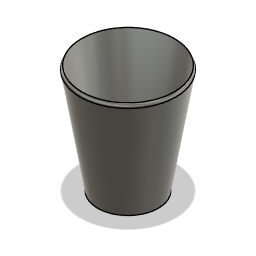
wzken爆改熔岩灯2顶盖刻字 (Autodesk Fusion 360 design; units mm, degrees)
Autodesk Fusion 360 part; units mm, degrees
(part 1 of 7)
sketch "草图1" plane through (0, 0, 0) normal (0, 1, 0) x (1, 0, 0)
  circle A0 centre (0, 0) radius 22.5
  circle A1 centre (0, 0) radius 13.75
  circle A2 centre (0, 0) radius 14.75
  circle A3 centre (0, 0) radius 23.5
  spline S0 degree 3 poles (1.8081, 3.6652) (1.7986, 3.6895) (1.7856, 3.712) (1.7795, 3.7138) knots 0 0 0 0 1 1 1 1
  dimension "d1" = 45
  dimension "d2" = 27.5
  dimension "d3" = 29.5
  dimension "d4" = 47
  constraint coincident A0.centre A1.centre
  constraint concentric A0 A1
  constraint concentric A0 A2
  constraint concentric A1 A3
  measures "d1" diameter of A0
  measures "d2" diameter of A1
  measures "d3" diameter of A2
  measures "d4" diameter of A3
extrude "拉伸1" add sketch "草图1" along normal blind 53 draft 9.4 contours A2
extrude "拉伸2" cut sketch "草图1" along normal blind 53 draft 9.4 contours A1
extrude "拉伸3" add sketch "草图1" along normal blind 2 draft 9.4 contours A1
fillet "圆角1" radius 2 1 edges at (-21.9322, 53, -8.5067)
sketch "草图2" plane through (0, 2, 0) normal (0, 1, 0) x (-1, 0, 0)
  circle A0 centre (0, 0) radius 14.0811
  line L0 (27.3607, -10.0098) -> (27.3607, 8.4871)
  line L1 (27.3607, 8.4871) -> (-0.3846, 8.4871)
  line L2 (-0.3846, 8.4871) -> (-28.1299, 8.4871)
  line L3 (-28.1299, 8.4871) -> (-28.1299, -10.0098)
  line L4 (-28.1299, -10.0098) -> (-28.1299, -28.5067)
  line L5 (-28.1299, -28.5067) -> (-0.3846, -28.5067)
  line L6 (-0.3846, -28.5067) -> (27.3607, -28.5067)
  line L7 (27.3607, -28.5067) -> (27.3607, -10.0098)
  spline S0 degree 3 poles (-1.1505, -12.3075) (-1.1794, -12.2641) (-1.1938, -11.6572) (-1.1866, -10.9708) knots 0 0 0 0 1 1 1 1
  line L8 (-1.1866, -10.9708) -> (-1.1721, -9.7136)
  line L9 (-1.1721, -9.7136) -> (-1.3455, -9.8292)
  spline S1 degree 3 poles (-1.3455, -9.8292) (-1.4395, -9.887) (-1.6707, -10.1326) (-1.8513, -10.3711) knots 0 0 0 0 1 1 1 1
  line L10 (-1.8513, -10.3711) -> (-2.1837, -10.7974)
  line L11 (-2.1837, -10.7974) -> (-1.9236, -10.819)
  spline S2 degree 3 poles (-1.9236, -10.819) (-1.7791, -10.8335) (-1.649, -10.8841) (-1.6273, -10.9347) knots 0 0 0 0 1 1 1 1
  spline S3 degree 3 poles (-1.6273, -10.9347) (-1.6056, -10.9997) (-1.7502, -11.0214) (-2.1837, -11.0214) knots 0 0 0 0 1 1 1 1
  spline S4 degree 3 poles (-2.1837, -11.0214) (-2.5088, -11.0214) (-2.7689, -10.9925) (-2.7689, -10.9563) knots 0 0 0 0 1 1 1 1
  spline S5 degree 3 poles (-2.7689, -10.9563) (-2.7689, -10.9202) (-2.5883, -10.7323) (-2.3715, -10.5517) knots 0 0 0 0 1 1 1 1
  spline S6 degree 3 poles (-2.3715, -10.5517) (-2.1548, -10.3639) (-1.9958, -10.1832) (-2.0175, -10.1471) knots 0 0 0 0 1 1 1 1
  spline S7 degree 3 poles (-2.0175, -10.1471) (-2.0392, -10.111) (-2.0175, -10.0893) (-1.9669, -10.0965) knots 0 0 0 0 1 1 1 1
  spline S8 degree 3 poles (-1.9669, -10.0965) (-1.9163, -10.111) (-1.8296, -10.0315) (-1.7646, -9.9231) knots 0 0 0 0 1 1 1 1
  spline S9 degree 3 poles (-1.7646, -9.9231) (-1.649, -9.728) (-1.649, -9.7208) (-2.1186, -9.2439) knots 0 0 0 0 1 1 1 1
  spline S10 degree 3 poles (-2.1186, -9.2439) (-2.3788, -8.9838) (-2.7183, -8.702) (-2.8773, -8.6153) knots 0 0 0 0 1 1 1 1
  line L12 (-2.8773, -8.6153) -> (-3.1663, -8.4564)
  line L13 (-3.1663, -8.4564) -> (-2.5955, -8.4347)
  spline S11 degree 3 poles (-2.5955, -8.4347) (-1.9814, -8.413) (-1.9091, -8.4347) (-2.0392, -8.5936) knots 0 0 0 0 1 1 1 1
  spline S12 degree 3 poles (-2.0392, -8.5936) (-2.1042, -8.6731) (-2.0319, -8.7743) (-1.6707, -9.1283) knots 0 0 0 0 1 1 1 1
  line L14 (-1.6707, -9.1283) -> (-1.2155, -9.5691)
  line L15 (-1.2155, -9.5691) -> (-1.1721, -9.3306)
  spline S13 degree 3 poles (-1.1721, -9.3306) (-1.0999, -8.8899) (-1.1721, -8.5936) (-1.3817, -8.5142) knots 0 0 0 0 1 1 1 1
  spline S14 degree 3 poles (-1.3817, -8.5142) (-1.5478, -8.4491) (-1.4756, -8.4347) (-0.9843, -8.4275) knots 0 0 0 0 1 1 1 1
  spline S15 degree 3 poles (-0.9843, -8.4275) (-0.399, -8.4202) (-0.1967, -8.4997) (-0.5652, -8.5936) knots 0 0 0 0 1 1 1 1
  line L16 (-0.5652, -8.5936) -> (-0.7458, -8.637)
  line L17 (-0.7458, -8.637) -> (-0.7314, -10.1326)
  line L18 (-0.7314, -10.1326) -> (-0.7097, -11.6283)
  line L19 (-0.7097, -11.6283) -> (-0.4279, -11.7078)
  spline S16 degree 3 poles (-0.4279, -11.7078) (-0.1245, -11.7945) (-0.1389, -11.8378) (-0.4929, -11.9173) knots 0 0 0 0 1 1 1 1
  spline S17 degree 3 poles (-0.4929, -11.9173) (-0.7675, -11.9896) (-0.8903, -12.0907) (-0.8903, -12.2569) knots 0 0 0 0 1 1 1 1
  spline S18 degree 3 poles (-0.8903, -12.2569) (-0.8903, -12.4086) (-1.071, -12.4447) (-1.1505, -12.3075) knots 0 0 0 0 1 1 1 1
  spline S19 degree 3 poles (5.5836, -11.6066) (5.5619, -11.5705) (5.6052, -11.5271) (5.6847, -11.5055) knots 0 0 0 0 1 1 1 1
  spline S20 degree 3 poles (5.6847, -11.5055) (5.8003, -11.4766) (5.8292, -11.4043) (5.8292, -11.1948) knots 0 0 0 0 1 1 1 1
  spline S21 degree 3 poles (5.8292, -11.1948) (5.8292, -10.9347) (5.3018, -9.2439) (5.1862, -9.1211) knots 0 0 0 0 1 1 1 1
  spline S22 degree 3 poles (5.1862, -9.1211) (5.1067, -9.0416) (4.8321, -9.6341) (4.7382, -10.0893) knots 0 0 0 0 1 1 1 1
  spline S23 degree 3 poles (4.7382, -10.0893) (4.6154, -10.6673) (4.8683, -11.491) (5.1934, -11.5416) knots 0 0 0 0 1 1 1 1
  spline S24 degree 3 poles (5.1934, -11.5416) (5.3524, -11.5705) (5.3451, -11.5777) (5.1573, -11.6283) knots 0 0 0 0 1 1 1 1
  spline S25 degree 3 poles (5.1573, -11.6283) (5.0489, -11.6644) (4.6732, -11.6644) (4.3264, -11.6355) knots 0 0 0 0 1 1 1 1
  spline S26 degree 3 poles (4.3264, -11.6355) (3.8206, -11.5922) (3.7339, -11.5705) (3.8784, -11.5127) knots 0 0 0 0 1 1 1 1
  spline S27 degree 3 poles (3.8784, -11.5127) (4.2324, -11.3826) (4.3191, -11.2381) (4.2686, -10.8841) knots 0 0 0 0 1 1 1 1
  spline S28 degree 3 poles (4.2686, -10.8841) (4.218, -10.5373) (3.9362, -9.6919) (3.7556, -9.3306) knots 0 0 0 0 1 1 1 1
  line L20 (3.7556, -9.3306) -> (3.6472, -9.1283)
  line L21 (3.6472, -9.1283) -> (3.5316, -9.2945)
  spline S29 degree 3 poles (3.5316, -9.2945) (3.4738, -9.3812) (3.2498, -9.9014) (3.0475, -10.4361) knots 0 0 0 0 1 1 1 1
  spline S30 degree 3 poles (3.0475, -10.4361) (2.6356, -11.5127) (2.6356, -11.5055) (3.1559, -11.5344) knots 0 0 0 0 1 1 1 1
  spline S31 degree 3 poles (3.1559, -11.5344) (3.4015, -11.5416) (3.4015, -11.5488) (3.0836, -11.6066) knots 0 0 0 0 1 1 1 1
  spline S32 degree 3 poles (3.0836, -11.6066) (2.903, -11.6355) (2.5128, -11.6644) (2.2166, -11.6644) knots 0 0 0 0 1 1 1 1
  line L22 (2.2166, -11.6644) -> (1.6747, -11.6716)
  line L23 (1.6747, -11.6716) -> (1.9564, -11.5055)
  spline S33 degree 3 poles (1.9564, -11.5055) (2.2527, -11.332) (2.5056, -10.8913) (3.3004, -9.1283) knots 0 0 0 0 1 1 1 1
  spline S34 degree 3 poles (3.3004, -9.1283) (3.5099, -8.6587) (3.705, -8.2757) (3.7339, -8.2757) knots 0 0 0 0 1 1 1 1
  spline S35 degree 3 poles (3.7339, -8.2757) (3.7628, -8.2757) (3.9073, -8.5431) (4.0518, -8.8754) knots 0 0 0 0 1 1 1 1
  spline S36 degree 3 poles (4.0518, -8.8754) (4.5431, -9.9881) (4.5648, -10.0026) (4.7454, -9.4173) knots 0 0 0 0 1 1 1 1
  spline S37 degree 3 poles (4.7454, -9.4173) (4.9116, -8.9043) (5.1862, -8.2757) (5.2512, -8.2757) knots 0 0 0 0 1 1 1 1
  spline S38 degree 3 poles (5.2512, -8.2757) (5.3307, -8.2757) (5.6414, -9.0055) (6.0388, -10.1399) knots 0 0 0 0 1 1 1 1
  spline S39 degree 3 poles (6.0388, -10.1399) (6.4289, -11.2742) (6.5662, -11.5271) (6.7541, -11.5271) knots 0 0 0 0 1 1 1 1
  spline S40 degree 3 poles (6.7541, -11.5271) (6.8624, -11.5271) (6.8624, -11.5416) (6.7685, -11.5994) knots 0 0 0 0 1 1 1 1
  spline S41 degree 3 poles (6.7685, -11.5994) (6.6312, -11.6861) (5.6341, -11.6933) (5.5836, -11.6066) knots 0 0 0 0 1 1 1 1
  spline S42 degree 3 poles (-4.3657, -11.0864) (-4.6692, -10.9852) (-4.9365, -10.7468) (-4.9365, -10.5878) knots 0 0 0 0 1 1 1 1
  spline S43 degree 3 poles (-4.9365, -10.5878) (-4.9365, -10.3422) (-4.6764, -10.2121) (-4.055, -10.1471) knots 0 0 0 0 1 1 1 1
  spline S44 degree 3 poles (-4.055, -10.1471) (-3.0218, -10.0315) (-3.0363, -10.0387) (-3.0868, -9.7208) knots 0 0 0 0 1 1 1 1
  spline S45 degree 3 poles (-3.0868, -9.7208) (-3.1952, -9.0127) (-3.4264, -8.8176) (-4.1128, -8.8249) knots 0 0 0 0 1 1 1 1
  spline S46 degree 3 poles (-4.1128, -8.8249) (-4.4308, -8.8249) (-4.6331, -8.8754) (-4.8209, -8.9838) knots 0 0 0 0 1 1 1 1
  spline S47 degree 3 poles (-4.8209, -8.9838) (-5.1388, -9.1717) (-5.1605, -9.085) (-4.8643, -8.796) knots 0 0 0 0 1 1 1 1
  spline S48 degree 3 poles (-4.8643, -8.796) (-4.4308, -8.3624) (-3.6504, -8.2974) (-3.1735, -8.6587) knots 0 0 0 0 1 1 1 1
  spline S49 degree 3 poles (-3.1735, -8.6587) (-2.6244, -9.085) (-2.4366, -10.0459) (-2.8267, -10.4795) knots 0 0 0 0 1 1 1 1
  spline S50 degree 3 poles (-2.8267, -10.4795) (-3.123, -10.819) (-3.3108, -10.9563) (-3.6143, -11.0647) knots 0 0 0 0 1 1 1 1
  spline S51 degree 3 poles (-3.6143, -11.0647) (-3.9539, -11.1803) (-4.055, -11.1875) (-4.3657, -11.0864) knots 0 0 0 0 1 1 1 1
  spline S52 degree 3 poles (-5.9842, -11.0214) (-5.9264, -10.8407) (-6.1359, -10.819) (-6.3527, -10.9852) knots 0 0 0 0 1 1 1 1
  spline S53 degree 3 poles (-6.3527, -10.9852) (-6.5333, -11.1225) (-7.0319, -11.1225) (-7.2342, -10.978) knots 0 0 0 0 1 1 1 1
  spline S54 degree 3 poles (-7.2342, -10.978) (-7.3859, -10.8769) (-7.3931, -10.819) (-7.3931, -9.8436) knots 0 0 0 0 1 1 1 1
  spline S55 degree 3 poles (-7.3931, -9.8436) (-7.3931, -9.0488) (-7.4148, -8.7815) (-7.5015, -8.6587) knots 0 0 0 0 1 1 1 1
  spline S56 degree 3 poles (-7.5015, -8.6587) (-7.5955, -8.5214) (-7.5955, -8.5069) (-7.4437, -8.4636) knots 0 0 0 0 1 1 1 1
  spline S57 degree 3 poles (-7.4437, -8.4636) (-7.227, -8.4058) (-6.7067, -8.4058) (-6.6489, -8.4708) knots 0 0 0 0 1 1 1 1
  spline S58 degree 3 poles (-6.6489, -8.4708) (-6.62, -8.4925) (-6.6851, -8.5936) (-6.7862, -8.6876) knots 0 0 0 0 1 1 1 1
  spline S59 degree 3 poles (-6.7862, -8.6876) (-6.9741, -8.861) (-6.9741, -8.8754) (-6.9452, -9.7208) knots 0 0 0 0 1 1 1 1
  spline S60 degree 3 poles (-6.9452, -9.7208) (-6.9235, -10.2844) (-6.8801, -10.6167) (-6.8223, -10.689) knots 0 0 0 0 1 1 1 1
  spline S61 degree 3 poles (-6.8223, -10.689) (-6.7212, -10.8118) (-6.4755, -10.8335) (-6.0998, -10.7612) knots 0 0 0 0 1 1 1 1
  line L24 (-6.0998, -10.7612) -> (-5.8758, -10.7179)
  line L25 (-5.8758, -10.7179) -> (-5.8758, -9.7136)
  line L26 (-5.8758, -9.7136) -> (-5.8758, -8.7093)
  line L27 (-5.8758, -8.7093) -> (-6.0781, -8.6225)
  line L28 (-6.0781, -8.6225) -> (-6.2732, -8.5431)
  line L29 (-6.2732, -8.5431) -> (-6.0565, -8.4853)
  spline S62 degree 3 poles (-6.0565, -8.4853) (-5.9408, -8.4491) (-5.6518, -8.4275) (-5.4206, -8.4347) knots 0 0 0 0 1 1 1 1
  line L30 (-5.4206, -8.4347) -> (-5.0016, -8.4419)
  line L31 (-5.0016, -8.4419) -> (-5.1894, -8.5936)
  spline S63 degree 3 poles (-5.1894, -8.5936) (-5.3773, -8.7454) (-5.3845, -8.7743) (-5.4206, -9.7352) knots 0 0 0 0 1 1 1 1
  line L32 (-5.4206, -9.7352) -> (-5.464, -10.7179)
  line L33 (-5.464, -10.7179) -> (-5.2544, -10.7468)
  line L34 (-5.2544, -10.7468) -> (-5.0449, -10.7685)
  line L35 (-5.0449, -10.7685) -> (-5.2833, -10.8985)
  spline S64 degree 3 poles (-5.2833, -10.8985) (-5.4134, -10.9708) (-5.5435, -11.0141) (-5.5724, -10.9925) knots 0 0 0 0 1 1 1 1
  spline S65 degree 3 poles (-5.5724, -10.9925) (-5.6013, -10.978) (-5.7024, -11.0069) (-5.8036, -11.0647) knots 0 0 0 0 1 1 1 1
  spline S66 degree 3 poles (-5.8036, -11.0647) (-6.0348, -11.1875) (-6.0348, -11.1875) (-5.9842, -11.0214) knots 0 0 0 0 1 1 1 1
  spline S67 degree 3 poles (-0.3484, -11.0286) (-0.3701, -10.9925) (-0.0667, -10.5589) (0.3235, -10.0676) knots 0 0 0 0 1 1 1 1
  spline S68 degree 3 poles (0.3235, -10.0676) (0.7137, -9.5763) (1.1255, -9.0561) (1.2339, -8.9116) knots 0 0 0 0 1 1 1 1
  line L36 (1.2339, -8.9116) -> (1.4362, -8.637)
  line L37 (1.4362, -8.637) -> (0.8654, -8.637)
  spline S69 degree 3 poles (0.8654, -8.637) (0.2151, -8.637) (0.0562, -8.7165) (-0.1678, -9.1283) knots 0 0 0 0 1 1 1 1
  spline S70 degree 3 poles (-0.1678, -9.1283) (-0.2906, -9.374) (-0.3051, -9.3812) (-0.3123, -9.215) knots 0 0 0 0 1 1 1 1
  spline S71 degree 3 poles (-0.3123, -9.215) (-0.3123, -9.1139) (-0.2545, -8.8971) (-0.1895, -8.7309) knots 0 0 0 0 1 1 1 1
  line L38 (-0.1895, -8.7309) -> (-0.0594, -8.4202)
  line L39 (-0.0594, -8.4202) -> (1.075, -8.4202)
  spline S72 degree 3 poles (1.075, -8.4202) (1.8914, -8.4202) (2.2166, -8.4419) (2.2166, -8.5069) knots 0 0 0 0 1 1 1 1
  spline S73 degree 3 poles (2.2166, -8.5069) (2.2166, -8.6153) (1.7469, -9.215) (1.0027, -10.0676) knots 0 0 0 0 1 1 1 1
  spline S74 degree 3 poles (1.0027, -10.0676) (0.3163, -10.8552) (0.3235, -10.8985) (1.0894, -10.8263) knots 0 0 0 0 1 1 1 1
  spline S75 degree 3 poles (1.0894, -10.8263) (1.5663, -10.7829) (1.5735, -10.7757) (1.7325, -10.4867) knots 0 0 0 0 1 1 1 1
  line L40 (1.7325, -10.4867) -> (1.8914, -10.1904)
  line L41 (1.8914, -10.1904) -> (1.9131, -10.4578)
  spline S76 degree 3 poles (1.9131, -10.4578) (1.9564, -10.978) (1.8914, -11.0141) (0.8943, -11.043) knots 0 0 0 0 1 1 1 1
  spline S77 degree 3 poles (0.8943, -11.043) (0.4102, -11.0503) (-0.0594, -11.0719) (-0.1461, -11.0792) knots 0 0 0 0 1 1 1 1
  spline S78 degree 3 poles (-0.1461, -11.0792) (-0.2328, -11.0864) (-0.3195, -11.0647) (-0.3484, -11.0286) knots 0 0 0 0 1 1 1 1
  spline S79 degree 3 poles (-3.3759, -10.7685) (-3.0507, -10.5734) (-2.8484, -10.2482) (-3.0146, -10.1832) knots 0 0 0 0 1 1 1 1
  spline S80 degree 3 poles (-3.0146, -10.1832) (-3.0652, -10.1615) (-3.2892, -10.1904) (-3.4987, -10.2555) knots 0 0 0 0 1 1 1 1
  spline S81 degree 3 poles (-3.4987, -10.2555) (-3.7154, -10.3133) (-4.0406, -10.3783) (-4.2357, -10.4072) knots 0 0 0 0 1 1 1 1
  spline S82 degree 3 poles (-4.2357, -10.4072) (-4.4235, -10.4289) (-4.5753, -10.465) (-4.5753, -10.4867) knots 0 0 0 0 1 1 1 1
  spline S83 degree 3 poles (-4.5753, -10.4867) (-4.5753, -10.5011) (-4.4886, -10.6167) (-4.3802, -10.7323) knots 0 0 0 0 1 1 1 1
  spline S84 degree 3 poles (-4.3802, -10.7323) (-4.1417, -11.0069) (-3.7949, -11.0214) (-3.3759, -10.7685) knots 0 0 0 0 1 1 1 1
extrude "拉伸4" cut sketch "草图2" against normal blind 1 contours S0 L8 L9 S1 L10 L11 S2 S3 S4 S5 S6 S7 S8 S9 S10 L12 L13 S11 S12 L14 L15 S13 S14 S15 L16 L17 L18 L19 S16 S17 S18 | S19 S20 S21 S22 S23 S24 S25 S26 S27 S28 L20 L21 S29 S30 S31 S32 L22 L23 S33 S34 S35 S36 S37 S38 S39 S40 S41 | S42 S43 S44 S45 S46 S47 S48 S49 S50 S51 | S52 S53 S54 S55 S56 S57 S58 S59 S60 S61 L24 L25 L26 L27 L28 L29 S62 L30 L31 S63 L32 L33 L34 L35 S64 S65 S66 | S67 S68 L36 L37 S69 S70 S71 L38 L39 S72 S73 S74 S75 L40 L41 S76 S77 S78
sketch "草图3" plane through (0, 2, 0) normal (0, 1, 0) x (-1, 0, 0)
  circle A0 centre (0, 0) radius 14.0811
  spline S0 degree 3 poles (-5.2833, -10.8985) (-5.4134, -10.9708) (-5.5435, -11.0141) (-5.5724, -10.9925) knots 0 0 0 0 1 1 1 1
  spline S1 degree 3 poles (-5.5724, -10.9925) (-5.6013, -10.978) (-5.7024, -11.0069) (-5.8036, -11.0647) knots 0 0 0 0 1 1 1 1
  spline S2 degree 3 poles (-5.8036, -11.0647) (-6.0348, -11.1875) (-6.0348, -11.1875) (-5.9842, -11.0214) knots 0 0 0 0 1 1 1 1
  spline S3 degree 3 poles (-5.9842, -11.0214) (-5.9264, -10.8407) (-6.1359, -10.819) (-6.3527, -10.9852) knots 0 0 0 0 1 1 1 1
  spline S4 degree 3 poles (-6.3527, -10.9852) (-6.5333, -11.1225) (-7.0319, -11.1225) (-7.2342, -10.978) knots 0 0 0 0 1 1 1 1
  spline S5 degree 3 poles (-7.2342, -10.978) (-7.3859, -10.8769) (-7.3931, -10.819) (-7.3931, -9.8436) knots 0 0 0 0 1 1 1 1
  spline S6 degree 3 poles (-7.3931, -9.8436) (-7.3931, -9.0488) (-7.4148, -8.7815) (-7.5015, -8.6587) knots 0 0 0 0 1 1 1 1
  spline S7 degree 3 poles (-7.5015, -8.6587) (-7.5955, -8.5214) (-7.5955, -8.5069) (-7.4437, -8.4636) knots 0 0 0 0 1 1 1 1
  spline S8 degree 3 poles (-7.4437, -8.4636) (-7.227, -8.4058) (-6.7067, -8.4058) (-6.6489, -8.4708) knots 0 0 0 0 1 1 1 1
  spline S9 degree 3 poles (-6.6489, -8.4708) (-6.62, -8.4925) (-6.6851, -8.5936) (-6.7862, -8.6876) knots 0 0 0 0 1 1 1 1
  spline S10 degree 3 poles (-6.7862, -8.6876) (-6.9741, -8.861) (-6.9741, -8.8754) (-6.9452, -9.7208) knots 0 0 0 0 1 1 1 1
  spline S11 degree 3 poles (-6.9452, -9.7208) (-6.9235, -10.2844) (-6.8801, -10.6167) (-6.8223, -10.689) knots 0 0 0 0 1 1 1 1
  spline S12 degree 3 poles (-6.8223, -10.689) (-6.7212, -10.8118) (-6.4755, -10.8335) (-6.0998, -10.7612) knots 0 0 0 0 1 1 1 1
  line L0 (-6.0998, -10.7612) -> (-5.8758, -10.7179)
  line L1 (-5.8758, -10.7179) -> (-5.8758, -8.7093)
  line L2 (-5.8758, -8.7093) -> (-6.0781, -8.6225)
  line L3 (-6.0781, -8.6225) -> (-6.2732, -8.5431)
  line L4 (-6.2732, -8.5431) -> (-6.0565, -8.4853)
  spline S13 degree 3 poles (-6.0565, -8.4853) (-5.9408, -8.4491) (-5.6518, -8.4275) (-5.4206, -8.4347) knots 0 0 0 0 1 1 1 1
  line L5 (-5.4206, -8.4347) -> (-5.0016, -8.4419)
  line L6 (-5.0016, -8.4419) -> (-5.1894, -8.5936)
  spline S14 degree 3 poles (-5.1894, -8.5936) (-5.3773, -8.7454) (-5.3845, -8.7743) (-5.4206, -9.7352) knots 0 0 0 0 1 1 1 1
  line L7 (-5.4206, -9.7352) -> (-5.464, -10.7179)
  line L8 (-5.464, -10.7179) -> (-5.2544, -10.7468)
  line L9 (-5.2544, -10.7468) -> (-5.0449, -10.7685)
  line L10 (-5.0449, -10.7685) -> (-5.2833, -10.8985)
  spline S15 degree 3 poles (6.0388, -10.1399) (6.4289, -11.2742) (6.5662, -11.5271) (6.7541, -11.5271) knots 0 0 0 0 1 1 1 1
  spline S16 degree 3 poles (6.7541, -11.5271) (6.8624, -11.5271) (6.8624, -11.5416) (6.7685, -11.5994) knots 0 0 0 0 1 1 1 1
  spline S17 degree 3 poles (6.7685, -11.5994) (6.6312, -11.6861) (5.6341, -11.6933) (5.5836, -11.6066) knots 0 0 0 0 1 1 1 1
  spline S18 degree 3 poles (5.5836, -11.6066) (5.5619, -11.5705) (5.6052, -11.5271) (5.6847, -11.5055) knots 0 0 0 0 1 1 1 1
  spline S19 degree 3 poles (5.6847, -11.5055) (5.8003, -11.4766) (5.8292, -11.4043) (5.8292, -11.1948) knots 0 0 0 0 1 1 1 1
  spline S20 degree 3 poles (5.8292, -11.1948) (5.8292, -10.9347) (5.3018, -9.2439) (5.1862, -9.1211) knots 0 0 0 0 1 1 1 1
  spline S21 degree 3 poles (5.1862, -9.1211) (5.1067, -9.0416) (4.8321, -9.6341) (4.7382, -10.0893) knots 0 0 0 0 1 1 1 1
  spline S22 degree 3 poles (4.7382, -10.0893) (4.6154, -10.6673) (4.8683, -11.491) (5.1934, -11.5416) knots 0 0 0 0 1 1 1 1
  spline S23 degree 3 poles (5.1934, -11.5416) (5.3524, -11.5705) (5.3451, -11.5777) (5.1573, -11.6283) knots 0 0 0 0 1 1 1 1
  spline S24 degree 3 poles (5.1573, -11.6283) (5.0489, -11.6644) (4.6732, -11.6644) (4.3264, -11.6355) knots 0 0 0 0 1 1 1 1
  spline S25 degree 3 poles (4.3264, -11.6355) (3.8206, -11.5922) (3.7339, -11.5705) (3.8784, -11.5127) knots 0 0 0 0 1 1 1 1
  spline S26 degree 3 poles (3.8784, -11.5127) (4.2324, -11.3826) (4.3191, -11.2381) (4.2686, -10.8841) knots 0 0 0 0 1 1 1 1
  spline S27 degree 3 poles (4.2686, -10.8841) (4.218, -10.5373) (3.9362, -9.6919) (3.7556, -9.3306) knots 0 0 0 0 1 1 1 1
  line L11 (3.7556, -9.3306) -> (3.6472, -9.1283)
  line L12 (3.6472, -9.1283) -> (3.5316, -9.2945)
  spline S28 degree 3 poles (3.5316, -9.2945) (3.4738, -9.3812) (3.2498, -9.9014) (3.0475, -10.4361) knots 0 0 0 0 1 1 1 1
  spline S29 degree 3 poles (3.0475, -10.4361) (2.6356, -11.5127) (2.6356, -11.5055) (3.1559, -11.5344) knots 0 0 0 0 1 1 1 1
  spline S30 degree 3 poles (3.1559, -11.5344) (3.4015, -11.5416) (3.4015, -11.5488) (3.0836, -11.6066) knots 0 0 0 0 1 1 1 1
  spline S31 degree 3 poles (3.0836, -11.6066) (2.903, -11.6355) (2.5128, -11.6644) (2.2166, -11.6644) knots 0 0 0 0 1 1 1 1
  line L13 (2.2166, -11.6644) -> (1.6747, -11.6716)
  line L14 (1.6747, -11.6716) -> (1.9564, -11.5055)
  spline S32 degree 3 poles (1.9564, -11.5055) (2.2527, -11.332) (2.5056, -10.8913) (3.3004, -9.1283) knots 0 0 0 0 1 1 1 1
  spline S33 degree 3 poles (3.3004, -9.1283) (3.5099, -8.6587) (3.705, -8.2757) (3.7339, -8.2757) knots 0 0 0 0 1 1 1 1
  spline S34 degree 3 poles (3.7339, -8.2757) (3.7628, -8.2757) (3.9073, -8.5431) (4.0518, -8.8754) knots 0 0 0 0 1 1 1 1
  spline S35 degree 3 poles (4.0518, -8.8754) (4.5431, -9.9881) (4.5648, -10.0026) (4.7454, -9.4173) knots 0 0 0 0 1 1 1 1
  spline S36 degree 3 poles (4.7454, -9.4173) (4.9116, -8.9043) (5.1862, -8.2757) (5.2512, -8.2757) knots 0 0 0 0 1 1 1 1
  spline S37 degree 3 poles (5.2512, -8.2757) (5.3307, -8.2757) (5.6414, -9.0055) (6.0388, -10.1399) knots 0 0 0 0 1 1 1 1
  spline S38 degree 3 poles (-3.1735, -8.6587) (-2.6244, -9.085) (-2.4366, -10.0459) (-2.8267, -10.4795) knots 0 0 0 0 1 1 1 1
  spline S39 degree 3 poles (-2.8267, -10.4795) (-3.123, -10.819) (-3.3108, -10.9563) (-3.6143, -11.0647) knots 0 0 0 0 1 1 1 1
  spline S40 degree 3 poles (-3.6143, -11.0647) (-3.9539, -11.1803) (-4.055, -11.1875) (-4.3657, -11.0864) knots 0 0 0 0 1 1 1 1
  spline S41 degree 3 poles (-4.3657, -11.0864) (-4.6692, -10.9852) (-4.9365, -10.7468) (-4.9365, -10.5878) knots 0 0 0 0 1 1 1 1
  spline S42 degree 3 poles (-4.9365, -10.5878) (-4.9365, -10.3422) (-4.6764, -10.2121) (-4.055, -10.1471) knots 0 0 0 0 1 1 1 1
  spline S43 degree 3 poles (-4.055, -10.1471) (-3.0218, -10.0315) (-3.0363, -10.0387) (-3.0868, -9.7208) knots 0 0 0 0 1 1 1 1
  spline S44 degree 3 poles (-3.0868, -9.7208) (-3.1952, -9.0127) (-3.4264, -8.8176) (-4.1128, -8.8249) knots 0 0 0 0 1 1 1 1
  spline S45 degree 3 poles (-4.1128, -8.8249) (-4.4308, -8.8249) (-4.6331, -8.8754) (-4.8209, -8.9838) knots 0 0 0 0 1 1 1 1
  spline S46 degree 3 poles (-4.8209, -8.9838) (-5.1388, -9.1717) (-5.1605, -9.085) (-4.8643, -8.796) knots 0 0 0 0 1 1 1 1
  spline S47 degree 3 poles (-4.8643, -8.796) (-4.4308, -8.3624) (-3.6504, -8.2974) (-3.1735, -8.6587) knots 0 0 0 0 1 1 1 1
  spline S48 degree 3 poles (1.9131, -10.4578) (1.9564, -10.978) (1.8914, -11.0141) (0.8943, -11.043) knots 0 0 0 0 1 1 1 1
  spline S49 degree 3 poles (0.8943, -11.043) (0.4102, -11.0503) (-0.0594, -11.0719) (-0.1461, -11.0792) knots 0 0 0 0 1 1 1 1
  spline S50 degree 3 poles (-0.1461, -11.0792) (-0.2328, -11.0864) (-0.3195, -11.0647) (-0.3484, -11.0286) knots 0 0 0 0 1 1 1 1
  spline S51 degree 3 poles (-0.3484, -11.0286) (-0.3701, -10.9925) (-0.0667, -10.5589) (0.3235, -10.0676) knots 0 0 0 0 1 1 1 1
  spline S52 degree 3 poles (0.3235, -10.0676) (0.7137, -9.5763) (1.1255, -9.0561) (1.2339, -8.9116) knots 0 0 0 0 1 1 1 1
  line L15 (1.2339, -8.9116) -> (1.4362, -8.637)
  line L16 (1.4362, -8.637) -> (0.8654, -8.637)
  spline S53 degree 3 poles (0.8654, -8.637) (0.2151, -8.637) (0.0562, -8.7165) (-0.1678, -9.1283) knots 0 0 0 0 1 1 1 1
  spline S54 degree 3 poles (-0.1678, -9.1283) (-0.2906, -9.374) (-0.3051, -9.3812) (-0.3123, -9.215) knots 0 0 0 0 1 1 1 1
  spline S55 degree 3 poles (-0.3123, -9.215) (-0.3123, -9.1139) (-0.2545, -8.8971) (-0.1895, -8.7309) knots 0 0 0 0 1 1 1 1
  line L17 (-0.1895, -8.7309) -> (-0.0594, -8.4202)
  line L18 (-0.0594, -8.4202) -> (1.075, -8.4202)
  spline S56 degree 3 poles (1.075, -8.4202) (1.8914, -8.4202) (2.2166, -8.4419) (2.2166, -8.5069) knots 0 0 0 0 1 1 1 1
  spline S57 degree 3 poles (2.2166, -8.5069) (2.2166, -8.6153) (1.7469, -9.215) (1.0027, -10.0676) knots 0 0 0 0 1 1 1 1
  spline S58 degree 3 poles (1.0027, -10.0676) (0.3163, -10.8552) (0.3235, -10.8985) (1.0894, -10.8263) knots 0 0 0 0 1 1 1 1
  spline S59 degree 3 poles (1.0894, -10.8263) (1.5663, -10.7829) (1.5735, -10.7757) (1.7325, -10.4867) knots 0 0 0 0 1 1 1 1
  line L19 (1.7325, -10.4867) -> (1.8914, -10.1904)
  line L20 (1.8914, -10.1904) -> (1.9131, -10.4578)
  spline S60 degree 3 poles (-0.4279, -11.7078) (-0.1245, -11.7945) (-0.1389, -11.8378) (-0.4929, -11.9173) knots 0 0 0 0 1 1 1 1
  spline S61 degree 3 poles (-0.4929, -11.9173) (-0.7675, -11.9896) (-0.8903, -12.0907) (-0.8903, -12.2569) knots 0 0 0 0 1 1 1 1
  spline S62 degree 3 poles (-0.8903, -12.2569) (-0.8903, -12.4086) (-1.071, -12.4447) (-1.1505, -12.3075) knots 0 0 0 0 1 1 1 1
  spline S63 degree 3 poles (-1.1505, -12.3075) (-1.1794, -12.2641) (-1.1938, -11.6572) (-1.1866, -10.9708) knots 0 0 0 0 1 1 1 1
  line L21 (-1.1866, -10.9708) -> (-1.1721, -9.7136)
  line L22 (-1.1721, -9.7136) -> (-1.3455, -9.8292)
  spline S64 degree 3 poles (-1.3455, -9.8292) (-1.4395, -9.887) (-1.6707, -10.1326) (-1.8513, -10.3711) knots 0 0 0 0 1 1 1 1
  line L23 (-1.8513, -10.3711) -> (-2.1837, -10.7974)
  line L24 (-2.1837, -10.7974) -> (-1.9236, -10.819)
  spline S65 degree 3 poles (-1.9236, -10.819) (-1.7791, -10.8335) (-1.649, -10.8841) (-1.6273, -10.9347) knots 0 0 0 0 1 1 1 1
  spline S66 degree 3 poles (-1.6273, -10.9347) (-1.6056, -10.9997) (-1.7502, -11.0214) (-2.1837, -11.0214) knots 0 0 0 0 1 1 1 1
  spline S67 degree 3 poles (-2.1837, -11.0214) (-2.5088, -11.0214) (-2.7689, -10.9925) (-2.7689, -10.9563) knots 0 0 0 0 1 1 1 1
  spline S68 degree 3 poles (-2.7689, -10.9563) (-2.7689, -10.9202) (-2.5883, -10.7323) (-2.3715, -10.5517) knots 0 0 0 0 1 1 1 1
  spline S69 degree 3 poles (-2.3715, -10.5517) (-2.1548, -10.3639) (-1.9958, -10.1832) (-2.0175, -10.1471) knots 0 0 0 0 1 1 1 1
  spline S70 degree 3 poles (-2.0175, -10.1471) (-2.0392, -10.111) (-2.0175, -10.0893) (-1.9669, -10.0965) knots 0 0 0 0 1 1 1 1
  spline S71 degree 3 poles (-1.9669, -10.0965) (-1.9163, -10.111) (-1.8296, -10.0315) (-1.7646, -9.9231) knots 0 0 0 0 1 1 1 1
  spline S72 degree 3 poles (-1.7646, -9.9231) (-1.649, -9.728) (-1.649, -9.7208) (-2.1186, -9.2439) knots 0 0 0 0 1 1 1 1
  spline S73 degree 3 poles (-2.1186, -9.2439) (-2.3788, -8.9838) (-2.7183, -8.702) (-2.8773, -8.6153) knots 0 0 0 0 1 1 1 1
  line L25 (-2.8773, -8.6153) -> (-3.1663, -8.4564)
  line L26 (-3.1663, -8.4564) -> (-2.5955, -8.4347)
  spline S74 degree 3 poles (-2.5955, -8.4347) (-1.9814, -8.413) (-1.9091, -8.4347) (-2.0392, -8.5936) knots 0 0 0 0 1 1 1 1
  spline S75 degree 3 poles (-2.0392, -8.5936) (-2.1042, -8.6731) (-2.0319, -8.7743) (-1.6707, -9.1283) knots 0 0 0 0 1 1 1 1
  line L27 (-1.6707, -9.1283) -> (-1.2155, -9.5691)
  line L28 (-1.2155, -9.5691) -> (-1.1721, -9.3306)
  spline S76 degree 3 poles (-1.1721, -9.3306) (-1.0999, -8.8899) (-1.1721, -8.5936) (-1.3817, -8.5142) knots 0 0 0 0 1 1 1 1
  spline S77 degree 3 poles (-1.3817, -8.5142) (-1.5478, -8.4491) (-1.4756, -8.4347) (-0.9843, -8.4275) knots 0 0 0 0 1 1 1 1
  spline S78 degree 3 poles (-0.9843, -8.4275) (-0.399, -8.4202) (-0.1967, -8.4997) (-0.5652, -8.5936) knots 0 0 0 0 1 1 1 1
  line L29 (-0.5652, -8.5936) -> (-0.7458, -8.637)
  line L30 (-0.7458, -8.637) -> (-0.7314, -10.1326)
  line L31 (-0.7314, -10.1326) -> (-0.7097, -11.6283)
  line L32 (-0.7097, -11.6283) -> (-0.4279, -11.7078)
  line L33 (-12.2434, 9.8661) -> (-12.2434, -2.3261)
  line L34 (-12.2434, -2.3261) -> (-0.0512, -2.3261)
  line L35 (-0.0512, -2.3261) -> (12.1411, -2.3261)
  line L36 (12.1411, -2.3261) -> (12.1411, 9.8661)
  line L37 (12.1411, 9.8661) -> (12.1411, 22.0584)
  line L38 (12.1411, 22.0584) -> (-0.0512, 22.0584)
  line L39 (-0.0512, 22.0584) -> (-12.2434, 22.0584)
  line L40 (-12.2434, 22.0584) -> (-12.2434, 9.8661)
  spline S79 degree 3 poles (2.5492, 13.4762) (2.5683, 13.4476) (2.5159, 13.3619) (2.4159, 13.2762) knots 0 0 0 0 1 1 1 1
  spline S80 degree 3 poles (2.4159, 13.2762) (2.2016, 13.0904) (1.3252, 12.4903) (1.0442, 12.3379) knots 0 0 0 0 1 1 1 1
  spline S81 degree 3 poles (1.0442, 12.3379) (0.9252, 12.276) (0.8014, 12.1951) (0.768, 12.1665) knots 0 0 0 0 1 1 1 1
  spline S82 degree 3 poles (0.768, 12.1665) (0.7347, 12.1331) (0.6728, 12.1046) (0.6299, 12.1046) knots 0 0 0 0 1 1 1 1
  spline S83 degree 3 poles (0.6299, 12.1046) (0.5918, 12.1046) (0.4775, 12.0331) (0.3775, 11.9474) knots 0 0 0 0 1 1 1 1
  spline S84 degree 3 poles (0.3775, 11.9474) (0.2727, 11.8617) (0.1298, 11.7569) (0.0584, 11.7188) knots 0 0 0 0 1 1 1 1
  spline S85 degree 3 poles (0.0584, 11.7188) (-0.0131, 11.6855) (-0.175, 11.5807) (-0.294, 11.4997) knots 0 0 0 0 1 1 1 1
  spline S86 degree 3 poles (-0.294, 11.4997) (-0.5417, 11.3235) (-0.637, 11.3045) (-0.6131, 11.4283) knots 0 0 0 0 1 1 1 1
  spline S87 degree 3 poles (-0.6131, 11.4283) (-0.5989, 11.514) (-0.5179, 11.5664) (0.4584, 12.176) knots 0 0 0 0 1 1 1 1
  spline S88 degree 3 poles (0.4584, 12.176) (0.7918, 12.3856) (1.2919, 12.7285) (1.5681, 12.9333) knots 0 0 0 0 1 1 1 1
  spline S89 degree 3 poles (1.5681, 12.9333) (2.0349, 13.2905) (2.4064, 13.5334) (2.4826, 13.5334) knots 0 0 0 0 1 1 1 1
  spline S90 degree 3 poles (2.4826, 13.5334) (2.5016, 13.5334) (2.5302, 13.5095) (2.5492, 13.4762) knots 0 0 0 0 1 1 1 1
  spline S91 degree 3 poles (0.9014, 11.0806) (0.9014, 10.5424) (0.9109, 10.1043) (0.9157, 10.1043) knots 0 0 0 0 1 1 1 1
  spline S92 degree 3 poles (0.9157, 10.1043) (0.9252, 10.1043) (1.049, 10.2186) (1.1919, 10.3567) knots 0 0 0 0 1 1 1 1
  spline S93 degree 3 poles (1.1919, 10.3567) (1.3348, 10.4948) (1.511, 10.6567) (1.5919, 10.7187) knots 0 0 0 0 1 1 1 1
  spline S94 degree 3 poles (1.5919, 10.7187) (1.7062, 10.8044) (1.7205, 10.833) (1.6634, 10.8711) knots 0 0 0 0 1 1 1 1
  spline S95 degree 3 poles (1.6634, 10.8711) (1.6253, 10.8949) (1.4967, 10.9092) (1.3776, 10.8996) knots 0 0 0 0 1 1 1 1
  spline S96 degree 3 poles (1.3776, 10.8996) (1.2157, 10.8949) (1.1633, 10.9092) (1.1633, 10.9615) knots 0 0 0 0 1 1 1 1
  spline S97 degree 3 poles (1.1633, 10.9615) (1.1633, 11.0187) (1.2633, 11.0377) (1.7015, 11.0473) knots 0 0 0 0 1 1 1 1
  spline S98 degree 3 poles (1.7015, 11.0473) (2.2349, 11.0616) (2.2397, 11.0568) (2.2254, 10.9568) knots 0 0 0 0 1 1 1 1
  spline S99 degree 3 poles (2.2254, 10.9568) (2.2158, 10.8853) (2.1349, 10.8091) (2.0063, 10.7425) knots 0 0 0 0 1 1 1 1
  spline S100 degree 3 poles (2.0063, 10.7425) (1.5919, 10.5234) (1.049, 10.009) (1.2347, 10.009) knots 0 0 0 0 1 1 1 1
  spline S101 degree 3 poles (1.2347, 10.009) (1.2633, 10.009) (1.2824, 9.9662) (1.2824, 9.9185) knots 0 0 0 0 1 1 1 1
  spline S102 degree 3 poles (1.2824, 9.9185) (1.2824, 9.8661) (1.3014, 9.8185) (1.3252, 9.809) knots 0 0 0 0 1 1 1 1
  spline S103 degree 3 poles (1.3252, 9.809) (1.3491, 9.8042) (1.4538, 9.6661) (1.5634, 9.5089) knots 0 0 0 0 1 1 1 1
  spline S104 degree 3 poles (1.5634, 9.5089) (1.8682, 9.0708) (2.0301, 8.9136) (2.1682, 8.9136) knots 0 0 0 0 1 1 1 1
  line L41 (2.1682, 8.9136) -> (2.292, 8.9136)
  line L42 (2.292, 8.9136) -> (2.1444, 9.0803)
  spline S105 degree 3 poles (2.1444, 9.0803) (2.0682, 9.1708) (1.9777, 9.3375) (1.9444, 9.447) knots 0 0 0 0 1 1 1 1
  spline S106 degree 3 poles (1.9444, 9.447) (1.8729, 9.7233) (1.9158, 10.1852) (2.0349, 10.4234) knots 0 0 0 0 1 1 1 1
  spline S107 degree 3 poles (2.0349, 10.4234) (2.1492, 10.6424) (2.6159, 11.0377) (2.8159, 11.0806) knots 0 0 0 0 1 1 1 1
  spline S108 degree 3 poles (2.8159, 11.0806) (3.1779, 11.1616) (3.6399, 10.8472) (3.8066, 10.4091) knots 0 0 0 0 1 1 1 1
  spline S109 degree 3 poles (3.8066, 10.4091) (3.8589, 10.2662) (3.9018, 10.1281) (3.9018, 10.1043) knots 0 0 0 0 1 1 1 1
  spline S110 degree 3 poles (3.9018, 10.1043) (3.9018, 10.0757) (3.5494, 10.0519) (3.0826, 10.0471) knots 0 0 0 0 1 1 1 1
  line L43 (3.0826, 10.0471) -> (2.2587, 10.0328)
  line L44 (2.2587, 10.0328) -> (2.2444, 9.8947)
  spline S111 degree 3 poles (2.2444, 9.8947) (2.2111, 9.628) (2.2825, 9.4423) (2.4826, 9.247) knots 0 0 0 0 1 1 1 1
  spline S112 degree 3 poles (2.4826, 9.247) (2.8493, 8.8993) (3.1207, 8.885) (3.5922, 9.1994) knots 0 0 0 0 1 1 1 1
  spline S113 degree 3 poles (3.5922, 9.1994) (3.9161, 9.4137) (3.9494, 9.4232) (3.9494, 9.3042) knots 0 0 0 0 1 1 1 1
  spline S114 degree 3 poles (3.9494, 9.3042) (3.9494, 9.1613) (3.6589, 8.8612) (3.4065, 8.7422) knots 0 0 0 0 1 1 1 1
  spline S115 degree 3 poles (3.4065, 8.7422) (3.1827, 8.6374) (3.1065, 8.6279) (2.3587, 8.6279) knots 0 0 0 0 1 1 1 1
  line L45 (2.3587, 8.6279) -> (1.5586, 8.6279)
  line L46 (1.5586, 8.6279) -> (1.5872, 8.7755)
  spline S116 degree 3 poles (1.5872, 8.7755) (1.611, 8.9041) (1.5777, 8.9755) (1.3252, 9.3089) knots 0 0 0 0 1 1 1 1
  spline S117 degree 3 poles (1.3252, 9.3089) (1.1633, 9.5232) (1.0252, 9.7233) (1.0109, 9.7566) knots 0 0 0 0 1 1 1 1
  spline S118 degree 3 poles (1.0109, 9.7566) (0.9442, 9.9281) (0.9014, 9.7709) (0.9014, 9.347) knots 0 0 0 0 1 1 1 1
  line L47 (0.9014, 9.347) -> (0.9014, 8.8708)
  line L48 (0.9014, 8.8708) -> (1.1062, 8.8565)
  spline S119 degree 3 poles (1.1062, 8.8565) (1.2681, 8.8469) (1.3062, 8.8231) (1.3062, 8.7469) knots 0 0 0 0 1 1 1 1
  spline S120 degree 3 poles (1.3062, 8.7469) (1.3062, 8.6517) (1.2729, 8.6517) (-0.4798, 8.6517) knots 0 0 0 0 1 1 1 1
  line L49 (-0.4798, 8.6517) -> (-2.2658, 8.6517)
  line L50 (-2.2658, 8.6517) -> (-2.2801, 8.7612)
  spline S121 degree 3 poles (-2.2801, 8.7612) (-2.2943, 8.866) (-2.2991, 8.866) (-2.4944, 8.7136) knots 0 0 0 0 1 1 1 1
  spline S122 degree 3 poles (-2.4944, 8.7136) (-2.6992, 8.5517) (-3.0611, 8.2516) (-3.5231, 7.8468) knots 0 0 0 0 1 1 1 1
  spline S123 degree 3 poles (-3.5231, 7.8468) (-3.6707, 7.7182) (-4.1851, 7.2229) (-4.6709, 6.7466) knots 0 0 0 0 1 1 1 1
  spline S124 degree 3 poles (-4.6709, 6.7466) (-5.5377, 5.8894) (-5.7663, 5.7131) (-5.7663, 5.9037) knots 0 0 0 0 1 1 1 1
  spline S125 degree 3 poles (-5.7663, 5.9037) (-5.7663, 5.956) (-5.5567, 6.1846) (-5.2519, 6.4704) knots 0 0 0 0 1 1 1 1
  spline S126 degree 3 poles (-5.2519, 6.4704) (-4.79, 6.9038) (-4.3661, 7.2753) (-2.742, 8.6993) knots 0 0 0 0 1 1 1 1
  spline S127 degree 3 poles (-2.742, 8.6993) (-2.442, 8.9612) (-2.0848, 9.3089) (-1.9467, 9.4708) knots 0 0 0 0 1 1 1 1
  spline S128 degree 3 poles (-1.9467, 9.4708) (-1.8086, 9.6328) (-1.4418, 10.0281) (-1.1323, 10.3567) knots 0 0 0 0 1 1 1 1
  spline S129 degree 3 poles (-1.1323, 10.3567) (-0.8275, 10.6805) (-0.575, 10.9711) (-0.575, 11.0044) knots 0 0 0 0 1 1 1 1
  spline S130 degree 3 poles (-0.575, 11.0044) (-0.575, 11.0377) (-0.7179, 11.0568) (-1.0132, 11.0568) knots 0 0 0 0 1 1 1 1
  spline S131 degree 3 poles (-1.0132, 11.0568) (-1.3513, 11.0568) (-1.4657, 11.0377) (-1.5371, 10.9758) knots 0 0 0 0 1 1 1 1
  spline S132 degree 3 poles (-1.5371, 10.9758) (-1.5847, 10.933) (-1.6704, 10.8758) (-1.7276, 10.8472) knots 0 0 0 0 1 1 1 1
  spline S133 degree 3 poles (-1.7276, 10.8472) (-1.7847, 10.8187) (-1.8752, 10.7044) (-1.9324, 10.5901) knots 0 0 0 0 1 1 1 1
  spline S134 degree 3 poles (-1.9324, 10.5901) (-2.0276, 10.3948) (-2.1467, 10.3186) (-2.1467, 10.4615) knots 0 0 0 0 1 1 1 1
  spline S135 degree 3 poles (-2.1467, 10.4615) (-2.1467, 10.4996) (-2.1229, 10.6329) (-2.0896, 10.7568) knots 0 0 0 0 1 1 1 1
  spline S136 degree 3 poles (-2.0896, 10.7568) (-2.061, 10.8853) (-2.0181, 11.0711) (-1.9943, 11.1711) knots 0 0 0 0 1 1 1 1
  line L51 (-1.9943, 11.1711) -> (-1.9467, 11.3568)
  line L52 (-1.9467, 11.3568) -> (-1.0465, 11.3283)
  spline S137 degree 3 poles (-1.0465, 11.3283) (-0.4988, 11.3092) (-0.1369, 11.3187) (-0.1226, 11.3473) knots 0 0 0 0 1 1 1 1
  spline S138 degree 3 poles (-0.1226, 11.3473) (-0.0893, 11.3997) (0.0012, 11.4045) (0.0822, 11.3473) knots 0 0 0 0 1 1 1 1
  spline S139 degree 3 poles (0.0822, 11.3473) (0.206, 11.2711) (0.0774, 11.0616) (-0.3464, 10.6424) knots 0 0 0 0 1 1 1 1
  spline S140 degree 3 poles (-0.3464, 10.6424) (-0.5798, 10.4138) (-1.0418, 9.9376) (-1.3704, 9.5899) knots 0 0 0 0 1 1 1 1
  line L53 (-1.3704, 9.5899) -> (-1.9705, 8.9612)
  line L54 (-1.9705, 8.9612) -> (-1.0227, 8.9708)
  line L55 (-1.0227, 8.9708) -> (-0.0797, 8.9851)
  line L56 (-0.0797, 8.9851) -> (-0.0369, 9.1756)
  spline S141 degree 3 poles (-0.0369, 9.1756) (0.0203, 9.4137) (0.025, 9.4185) (0.1155, 9.328) knots 0 0 0 0 1 1 1 1
  spline S142 degree 3 poles (0.1155, 9.328) (0.1584, 9.2851) (0.187, 9.1708) (0.187, 9.0565) knots 0 0 0 0 1 1 1 1
  spline S143 degree 3 poles (0.187, 9.0565) (0.187, 8.866) (0.1917, 8.8612) (0.3394, 8.8755) knots 0 0 0 0 1 1 1 1
  spline S144 degree 3 poles (0.3394, 8.8755) (0.4727, 8.8898) (0.4965, 8.9136) (0.5299, 9.0565) knots 0 0 0 0 1 1 1 1
  spline S145 degree 3 poles (0.5299, 9.0565) (0.5727, 9.247) (0.5775, 10.8377) (0.5346, 11.2854) knots 0 0 0 0 1 1 1 1
  spline S146 degree 3 poles (0.5346, 11.2854) (0.5108, 11.5521) (0.4965, 11.595) (0.387, 11.6331) knots 0 0 0 0 1 1 1 1
  spline S147 degree 3 poles (0.387, 11.6331) (0.2679, 11.6807) (0.2727, 11.6807) (0.5489, 11.8664) knots 0 0 0 0 1 1 1 1
  spline S148 degree 3 poles (0.5489, 11.8664) (0.7013, 11.9712) (0.8442, 12.0569) (0.868, 12.0569) knots 0 0 0 0 1 1 1 1
  spline S149 degree 3 poles (0.868, 12.0569) (0.8871, 12.0569) (0.9014, 11.6188) (0.9014, 11.0806) knots 0 0 0 0 1 1 1 1
  spline S150 degree 3 poles (-1.8705, 11.795) (-1.68, 11.7474) (-1.7514, 11.6378) (-1.9895, 11.6045) knots 0 0 0 0 1 1 1 1
  spline S151 degree 3 poles (-1.9895, 11.6045) (-2.2229, 11.5712) (-2.4801, 11.4045) (-2.4801, 11.2806) knots 0 0 0 0 1 1 1 1
  spline S152 degree 3 poles (-2.4801, 11.2806) (-2.4801, 11.2473) (-2.4991, 11.1997) (-2.5229, 11.1759) knots 0 0 0 0 1 1 1 1
  spline S153 degree 3 poles (-2.5229, 11.1759) (-2.5468, 11.1473) (-2.7182, 10.7949) (-2.8992, 10.39) knots 0 0 0 0 1 1 1 1
  spline S154 degree 3 poles (-2.8992, 10.39) (-3.2373, 9.6423) (-3.8279, 8.4659) (-3.9184, 8.3516) knots 0 0 0 0 1 1 1 1
  spline S155 degree 3 poles (-3.9184, 8.3516) (-3.9946, 8.2659) (-4.0279, 8.3135) (-4.2137, 8.7803) knots 0 0 0 0 1 1 1 1
  spline S156 degree 3 poles (-4.2137, 8.7803) (-4.3042, 9.0089) (-4.4423, 9.3137) (-4.5185, 9.4661) knots 0 0 0 0 1 1 1 1
  line L57 (-4.5185, 9.4661) -> (-4.6566, 9.7376)
  line L58 (-4.6566, 9.7376) -> (-4.7947, 9.4089)
  spline S157 degree 3 poles (-4.7947, 9.4089) (-4.8709, 9.228) (-4.9471, 9.0755) (-4.9662, 9.066) knots 0 0 0 0 1 1 1 1
  spline S158 degree 3 poles (-4.9662, 9.066) (-4.99, 9.0565) (-5.0043, 9.0232) (-5.0043, 8.9898) knots 0 0 0 0 1 1 1 1
  spline S159 degree 3 poles (-5.0043, 8.9898) (-5.0043, 8.8946) (-5.2091, 8.4183) (-5.2662, 8.3802) knots 0 0 0 0 1 1 1 1
  spline S160 degree 3 poles (-5.2662, 8.3802) (-5.3424, 8.3278) (-5.4091, 8.4326) (-5.552, 8.8184) knots 0 0 0 0 1 1 1 1
  spline S161 degree 3 poles (-5.552, 8.8184) (-5.7091, 9.2375) (-6.0187, 9.9804) (-6.2616, 10.4996) knots 0 0 0 0 1 1 1 1
  spline S162 degree 3 poles (-6.2616, 10.4996) (-6.3569, 10.6996) (-6.4331, 10.8806) (-6.4331, 10.8949) knots 0 0 0 0 1 1 1 1
  spline S163 degree 3 poles (-6.4331, 10.8949) (-6.4331, 10.9758) (-6.695, 11.5188) (-6.7617, 11.5712) knots 0 0 0 0 1 1 1 1
  spline S164 degree 3 poles (-6.7617, 11.5712) (-6.7998, 11.5997) (-6.895, 11.6283) (-6.9712, 11.6283) knots 0 0 0 0 1 1 1 1
  spline S165 degree 3 poles (-6.9712, 11.6283) (-7.057, 11.6283) (-7.0998, 11.6474) (-7.0903, 11.6902) knots 0 0 0 0 1 1 1 1
  spline S166 degree 3 poles (-7.0903, 11.6902) (-7.076, 11.7283) (-6.9093, 11.7521) (-6.5331, 11.7617) knots 0 0 0 0 1 1 1 1
  spline S167 degree 3 poles (-6.5331, 11.7617) (-6.0425, 11.7712) (-5.9997, 11.7664) (-6.0139, 11.6902) knots 0 0 0 0 1 1 1 1
  spline S168 degree 3 poles (-6.0139, 11.6902) (-6.0235, 11.6378) (-6.0854, 11.595) (-6.1711, 11.5807) knots 0 0 0 0 1 1 1 1
  spline S169 degree 3 poles (-6.1711, 11.5807) (-6.2473, 11.5664) (-6.3045, 11.5426) (-6.2997, 11.5235) knots 0 0 0 0 1 1 1 1
  spline S170 degree 3 poles (-6.2997, 11.5235) (-6.2521, 11.3711) (-6.214, 11.2806) (-6.0901, 11.0092) knots 0 0 0 0 1 1 1 1
  spline S171 degree 3 poles (-6.0901, 11.0092) (-6.0092, 10.8377) (-5.8806, 10.552) (-5.8044, 10.3662) knots 0 0 0 0 1 1 1 1
  spline S172 degree 3 poles (-5.8044, 10.3662) (-5.7282, 10.1852) (-5.6377, 9.99) (-5.6044, 9.9376) knots 0 0 0 0 1 1 1 1
  spline S173 degree 3 poles (-5.6044, 9.9376) (-5.571, 9.8852) (-5.5043, 9.7376) (-5.4615, 9.6042) knots 0 0 0 0 1 1 1 1
  spline S174 degree 3 poles (-5.4615, 9.6042) (-5.4186, 9.4756) (-5.3519, 9.3137) (-5.3186, 9.2518) knots 0 0 0 0 1 1 1 1
  line L59 (-5.3186, 9.2518) -> (-5.2519, 9.1327)
  line L60 (-5.2519, 9.1327) -> (-5.1614, 9.3232)
  spline S175 degree 3 poles (-5.1614, 9.3232) (-5.109, 9.4232) (-5.0281, 9.609) (-4.9852, 9.728) knots 0 0 0 0 1 1 1 1
  spline S176 degree 3 poles (-4.9852, 9.728) (-4.9043, 9.9423) (-4.9043, 9.9566) (-5.0043, 10.2043) knots 0 0 0 0 1 1 1 1
  spline S177 degree 3 poles (-5.0043, 10.2043) (-5.1948, 10.6663) (-5.2519, 10.7901) (-5.3615, 11.0092) knots 0 0 0 0 1 1 1 1
  spline S178 degree 3 poles (-5.3615, 11.0092) (-5.4186, 11.1282) (-5.4853, 11.2902) (-5.4996, 11.3759) knots 0 0 0 0 1 1 1 1
  spline S179 degree 3 poles (-5.4996, 11.3759) (-5.5377, 11.5426) (-5.5996, 11.6093) (-5.7377, 11.6331) knots 0 0 0 0 1 1 1 1
  spline S180 degree 3 poles (-5.7377, 11.6331) (-5.7901, 11.6426) (-5.8377, 11.6807) (-5.852, 11.714) knots 0 0 0 0 1 1 1 1
  spline S181 degree 3 poles (-5.852, 11.714) (-5.8663, 11.7569) (-5.7425, 11.7712) (-5.3377, 11.7712) knots 0 0 0 0 1 1 1 1
  spline S182 degree 3 poles (-5.3377, 11.7712) (-4.8566, 11.7712) (-4.809, 11.7617) (-4.8233, 11.6902) knots 0 0 0 0 1 1 1 1
  spline S183 degree 3 poles (-4.8233, 11.6902) (-4.8328, 11.6378) (-4.8947, 11.595) (-4.9805, 11.5807) knots 0 0 0 0 1 1 1 1
  spline S184 degree 3 poles (-4.9805, 11.5807) (-5.0567, 11.5664) (-5.1281, 11.5235) (-5.1376, 11.4807) knots 0 0 0 0 1 1 1 1
  spline S185 degree 3 poles (-5.1376, 11.4807) (-5.1424, 11.4426) (-5.0757, 11.2425) (-4.9805, 11.0377) knots 0 0 0 0 1 1 1 1
  spline S186 degree 3 poles (-4.9805, 11.0377) (-4.89, 10.8377) (-4.8138, 10.6472) (-4.8138, 10.6186) knots 0 0 0 0 1 1 1 1
  spline S187 degree 3 poles (-4.8138, 10.6186) (-4.8138, 10.5281) (-4.6614, 10.2472) (-4.6233, 10.271) knots 0 0 0 0 1 1 1 1
  spline S188 degree 3 poles (-4.6233, 10.271) (-4.5566, 10.3091) (-4.3851, 10.7187) (-4.3851, 10.8282) knots 0 0 0 0 1 1 1 1
  spline S189 degree 3 poles (-4.3851, 10.8282) (-4.3899, 10.8901) (-4.428, 11.0235) (-4.4804, 11.1282) knots 0 0 0 0 1 1 1 1
  spline S190 degree 3 poles (-4.4804, 11.1282) (-4.5328, 11.233) (-4.5709, 11.3664) (-4.5756, 11.4283) knots 0 0 0 0 1 1 1 1
  spline S191 degree 3 poles (-4.5756, 11.4283) (-4.5756, 11.4854) (-4.609, 11.5473) (-4.6471, 11.5616) knots 0 0 0 0 1 1 1 1
  spline S192 degree 3 poles (-4.6471, 11.5616) (-4.6852, 11.5807) (-4.7185, 11.6331) (-4.7185, 11.6807) knots 0 0 0 0 1 1 1 1
  spline S193 degree 3 poles (-4.7185, 11.6807) (-4.7185, 11.7664) (-4.6757, 11.7712) (-4.1708, 11.7712) knots 0 0 0 0 1 1 1 1
  spline S194 degree 3 poles (-4.1708, 11.7712) (-3.6803, 11.7712) (-3.6231, 11.7617) (-3.6231, 11.6902) knots 0 0 0 0 1 1 1 1
  spline S195 degree 3 poles (-3.6231, 11.6902) (-3.6231, 11.6188) (-3.666, 11.6045) (-3.9041, 11.6045) knots 0 0 0 0 1 1 1 1
  spline S196 degree 3 poles (-3.9041, 11.6045) (-4.0613, 11.6045) (-4.2042, 11.5854) (-4.2232, 11.5664) knots 0 0 0 0 1 1 1 1
  spline S197 degree 3 poles (-4.2232, 11.5664) (-4.247, 11.5473) (-4.2327, 11.4616) (-4.1994, 11.3759) knots 0 0 0 0 1 1 1 1
  spline S198 degree 3 poles (-4.1994, 11.3759) (-4.1661, 11.2902) (-4.066, 11.033) (-3.9803, 10.7949) knots 0 0 0 0 1 1 1 1
  spline S199 degree 3 poles (-3.9803, 10.7949) (-3.8946, 10.5615) (-3.7565, 10.2186) (-3.6755, 10.0376) knots 0 0 0 0 1 1 1 1
  spline S200 degree 3 poles (-3.6755, 10.0376) (-3.5279, 9.7137) (-3.5231, 9.709) (-3.4517, 9.8138) knots 0 0 0 0 1 1 1 1
  spline S201 degree 3 poles (-3.4517, 9.8138) (-3.4088, 9.8709) (-3.2945, 10.1138) (-3.1945, 10.3567) knots 0 0 0 0 1 1 1 1
  spline S202 degree 3 poles (-3.1945, 10.3567) (-3.0945, 10.5996) (-2.9468, 10.9473) (-2.8659, 11.1282) knots 0 0 0 0 1 1 1 1
  spline S203 degree 3 poles (-2.8659, 11.1282) (-2.6658, 11.5807) (-2.6706, 11.6283) (-2.9087, 11.6283) knots 0 0 0 0 1 1 1 1
  spline S204 degree 3 poles (-2.9087, 11.6283) (-3.0564, 11.6283) (-3.0992, 11.6474) (-3.0992, 11.714) knots 0 0 0 0 1 1 1 1
  spline S205 degree 3 poles (-3.0992, 11.714) (-3.0992, 11.7855) (-3.0325, 11.795) (-2.5372, 11.8093) knots 0 0 0 0 1 1 1 1
  spline S206 degree 3 poles (-2.5372, 11.8093) (-2.2324, 11.8141) (-1.9324, 11.8093) (-1.8705, 11.795) knots 0 0 0 0 1 1 1 1
  spline S207 degree 3 poles (5.7878, 11.0282) (5.8783, 10.9854) (6.0164, 10.8711) (6.0926, 10.7758) knots 0 0 0 0 1 1 1 1
  line L61 (6.0926, 10.7758) -> (6.2355, 10.6043)
  line L62 (6.2355, 10.6043) -> (6.2403, 9.8423)
  spline S208 degree 3 poles (6.2403, 9.8423) (6.245, 8.9136) (6.2593, 8.8469) (6.4641, 8.8279) knots 0 0 0 0 1 1 1 1
  spline S209 degree 3 poles (6.4641, 8.8279) (6.5784, 8.8184) (6.6165, 8.7898) (6.6165, 8.7184) knots 0 0 0 0 1 1 1 1
  spline S210 degree 3 poles (6.6165, 8.7184) (6.6165, 8.6326) (6.5784, 8.6279) (6.045, 8.6279) knots 0 0 0 0 1 1 1 1
  spline S211 degree 3 poles (6.045, 8.6279) (5.7307, 8.6279) (5.4735, 8.6422) (5.4735, 8.666) knots 0 0 0 0 1 1 1 1
  spline S212 degree 3 poles (5.4735, 8.666) (5.4782, 8.7565) (5.5592, 8.8136) (5.7116, 8.8279) knots 0 0 0 0 1 1 1 1
  line L63 (5.7116, 8.8279) -> (5.8783, 8.8422)
  line L64 (5.8783, 8.8422) -> (5.8783, 9.6899)
  spline S213 degree 3 poles (5.8783, 9.6899) (5.8783, 10.4519) (5.8688, 10.5424) (5.7973, 10.5853) knots 0 0 0 0 1 1 1 1
  spline S214 degree 3 poles (5.7973, 10.5853) (5.7497, 10.6139) (5.7116, 10.6615) (5.7116, 10.6996) knots 0 0 0 0 1 1 1 1
  spline S215 degree 3 poles (5.7116, 10.6996) (5.7116, 10.7806) (5.4068, 10.8853) (5.2592, 10.8472) knots 0 0 0 0 1 1 1 1
  spline S216 degree 3 poles (5.2592, 10.8472) (5.202, 10.833) (5.0591, 10.7615) (4.9543, 10.6901) knots 0 0 0 0 1 1 1 1
  line L65 (4.9543, 10.6901) -> (4.7591, 10.5615)
  line L66 (4.7591, 10.5615) -> (4.7686, 9.7042)
  line L67 (4.7686, 9.7042) -> (4.7829, 8.8422)
  line L68 (4.7829, 8.8422) -> (4.9258, 8.8279)
  spline S217 degree 3 poles (4.9258, 8.8279) (5.0687, 8.8088) (5.1544, 8.7374) (5.1115, 8.666) knots 0 0 0 0 1 1 1 1
  spline S218 degree 3 poles (5.1115, 8.666) (5.0877, 8.6279) (3.9494, 8.6088) (3.9494, 8.6469) knots 0 0 0 0 1 1 1 1
  spline S219 degree 3 poles (3.9494, 8.6469) (3.9494, 8.7565) (4.0304, 8.8184) (4.1638, 8.8184) knots 0 0 0 0 1 1 1 1
  spline S220 degree 3 poles (4.1638, 8.8184) (4.2638, 8.8184) (4.3304, 8.8469) (4.3495, 8.8946) knots 0 0 0 0 1 1 1 1
  spline S221 degree 3 poles (4.3495, 8.8946) (4.3876, 8.9946) (4.3876, 10.4805) (4.3495, 10.671) knots 0 0 0 0 1 1 1 1
  spline S222 degree 3 poles (4.3495, 10.671) (4.3257, 10.7853) (4.2876, 10.8282) (4.178, 10.8568) knots 0 0 0 0 1 1 1 1
  spline S223 degree 3 poles (4.178, 10.8568) (3.8875, 10.9282) (4.0637, 11.0425) (4.4876, 11.052) knots 0 0 0 0 1 1 1 1
  spline S224 degree 3 poles (4.4876, 11.052) (4.6924, 11.0568) (4.7115, 11.0473) (4.7115, 10.9425) knots 0 0 0 0 1 1 1 1
  spline S225 degree 3 poles (4.7115, 10.9425) (4.7115, 10.7758) (4.7972, 10.7425) (4.9162, 10.8568) knots 0 0 0 0 1 1 1 1
  spline S226 degree 3 poles (4.9162, 10.8568) (5.183, 11.1044) (5.4973, 11.1663) (5.7878, 11.0282) knots 0 0 0 0 1 1 1 1
  spline S227 degree 3 poles (2.654, 10.8568) (2.5254, 10.8139) (2.3873, 10.5901) (2.3683, 10.3853) knots 0 0 0 0 1 1 1 1
  spline S228 degree 3 poles (2.3683, 10.3853) (2.354, 10.271) (2.354, 10.271) (2.8302, 10.29) knots 0 0 0 0 1 1 1 1
  spline S229 degree 3 poles (2.8302, 10.29) (3.0922, 10.2948) (3.316, 10.3138) (3.3255, 10.3234) knots 0 0 0 0 1 1 1 1
  spline S230 degree 3 poles (3.3255, 10.3234) (3.3636, 10.3567) (3.235, 10.7139) (3.1636, 10.771) knots 0 0 0 0 1 1 1 1
  spline S231 degree 3 poles (3.1636, 10.771) (3.0588, 10.8568) (2.7969, 10.9044) (2.654, 10.8568) knots 0 0 0 0 1 1 1 1
  spline S232 degree 3 poles (-4.2708, 10.3615) (-4.2851, 10.3138) (-4.3185, 10.2138) (-4.347, 10.1424) knots 0 0 0 0 1 1 1 1
  spline S233 degree 3 poles (-4.347, 10.1424) (-4.3708, 10.0757) (-4.3804, 9.9662) (-4.3613, 9.9042) knots 0 0 0 0 1 1 1 1
  spline S234 degree 3 poles (-4.3613, 9.9042) (-4.3089, 9.7185) (-3.9898, 9.0565) (-3.9565, 9.0565) knots 0 0 0 0 1 1 1 1
  spline S235 degree 3 poles (-3.9565, 9.0565) (-3.9374, 9.0565) (-3.8993, 9.1375) (-3.866, 9.2375) knots 0 0 0 0 1 1 1 1
  spline S236 degree 3 poles (-3.866, 9.2375) (-3.8089, 9.4042) (-3.8184, 9.447) (-4.0041, 9.9138) knots 0 0 0 0 1 1 1 1
  spline S237 degree 3 poles (-4.0041, 9.9138) (-4.1137, 10.19) (-4.2137, 10.4234) (-4.2232, 10.4329) knots 0 0 0 0 1 1 1 1
  spline S238 degree 3 poles (-4.2232, 10.4329) (-4.2327, 10.4424) (-4.2518, 10.4091) (-4.2708, 10.3615) knots 0 0 0 0 1 1 1 1
extrude "拉伸5" cut sketch "草图3" against normal blind 1 contours S79 S80 S81 S82 S83 S84 S85 S86 S87 S88 S89 S90 | S91 S92 S93 S94 S95 S96 S97 S98 S99 S100 S101 S102 S103 S104 L41 L42 S105 S106 S107 S108 S109 S110 L43 L44 S111 S112 S113 S114 S115 L45 L46 S116 S117 S118 L47 L48 S119 S120 L49 L50 S121 S122 S123 S124 S125 S126 S127 S128 S129 S130 S131 S132 S133 S134 S135 S136 L51 L52 S137 S138 S139 S140 L53 L54 L55 L56 S141 S142 S143 S144 S145 S146 S147 S148 S149 | S150 S151 S152 S153 S154 S155 S156 L57 L58 S157 S158 S159 S160 S161 S162 S163 S164 S165 S166 S167 S168 S169 S170 S171 S172 S173 S174 L59 L60 S175 S176 S177 S178 S179 S180 S181 S182 S183 S184 S185 S186 S187 S188 S189 S190 S191 S192 S193 S194 S195 S196 S197 S198 S199 S200 S201 S202 S203 S204 S205 S206 | S207 L61 L62 S208 S209 S210 S211 S212 L63 L64 S213 S214 S215 S216 L65 L66 L67 L68 S217 S218 S219 S220 S221 S222 S223 S224 S225 S226